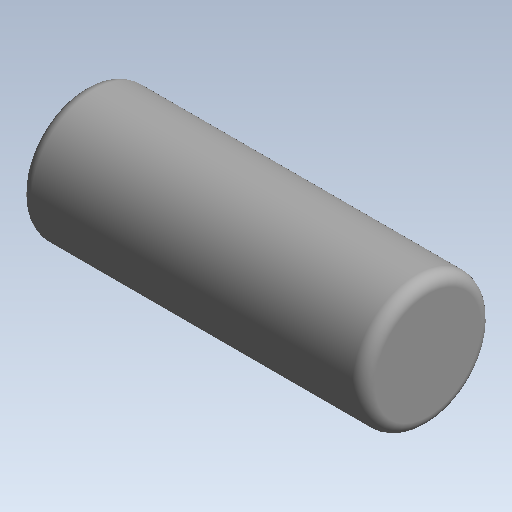
# Autodesk Inventor part: HK0408FT2RO
Saved by Autodesk Inventor 2021.3 (Build 253353010, 353A)
## iProperties
Category: PARTsolutions
Company: NTN
Part Number: HK0408FT2RO
Material: 一般
Catalog Web Link: www.cadenas.de
Description: Needle Roller Shell Bearings open-ended RO-
Vendor: NTN
Document SubType Name: Modeling
Designer: partserver
Manufacturer: NTN
Mass: 0.00703405 g
Surface Area: 0.218287 cm^2
Volume: 0.00703405 cm^3
Density: 1 g/cm^3
Appearance: PSOLRGB-192-192-192
PSOL_IDENT_0: {$CADENAS_DATA\23d-libs\ntn\needle_roler_bearings\needle_roller_shell_bearings_open_ended_ro.prj},19
PSOL_IDENT_1: 8 {VTYP=3D},{NB=HK0408FT2RO},{LINA=HK0408FT2RO},{NN=Needle Roller Shell Bearings open-ended RO},{DAT
PSOL_IDENT_2: E=23.10.2020 01:12:34},{GEOMDATE=20.04.2020 08:34:27},{VERSION=},{LINEID=20},{WBVAR=},{WBNUMERIC=}
PSOL_IDENT_3: {NB=HK0408FT2RO},{LINA=HK0408FT2RO},{KT=DUMMY},{FW=4},{D=8.0},{C=8},{ORDER=HK0408FT2},{CR=1770},{COR=
PSOL_IDENT_4: 1270},{CRF=180},{CORF=129},{LSG=30000},{LSO=45000},{MASS=0.0016},{IT=-},{RT=1.6},{VER=1},{T=0.500},{
PSOL_IDENT_5: DW=1.500},{LW=4.000},{NR=6.000},{CID=4.750},{CD=6.250},{CW=6.600},{SD=4.200}
NB: HK0408FT2RO
NN: Needle Roller Shell Bearings open-ended RO
NBSYN: $ORDER.RO
LINA: HK0408FT2RO
CATALOG: NTN Corporation
FW: 4
D: 8
C: 8
ORDER: HK0408FT2
CR: 1770
COR: 1270
CRF: 180
CORF: 129
LSG: 30000
LSO: 45000
MASS: 0.0016
IT: -
RT: 1.6
VER: 1
SUPPLIER: NTN
ARTICLENO: HK0408FT2RO
BOMINFO: HK0408FT2RO
CREATOR: CADENAS GmbH
Title: HK0408FT2RO
Author: Cadenas PARTsolutions
Autodesk Inventor part; units mm, degrees
sketch "Sketch_1" plane through (0, 0, 0) normal (0, 0, 1) x (1, 0, 0)
  line L0 (2, 0) -> (-2, 0)
  line L1 (-2, 0) -> (-2, 0.6167)
  arc A0 (-1.8667, 0.75) -> (-2, 0.6167) centre (-1.8667, 0.6167) ccw
  line L2 (-1.8667, 0.75) -> (1.8667, 0.75)
  arc A1 (2, 0.6167) -> (1.8667, 0.75) centre (1.8667, 0.6167) ccw
  line L3 (2, 0.6167) -> (2, 0)
  line L4 (2, 0) -> (-2, 0)
  constraints: 10 end point, 4 point on circle, 2 centre point
revolve "Revolution1" add sketch "Sketch_1" angle 360 about axis through (2, 0, 0) along (1, 0, 0)
ref_plane "IP_1_XY" through (0, 0, 0) normal (1, 0, 0) x (0, 0, -1)
ref_plane "IP_1_YZ" through (0, 0, 0) normal (0, 0, -1) x (0, 1, 0)
ref_plane "IP_1_ZX" through (0, 0, 0) normal (0, 1, 0) x (1, 0, 0)
body "Solid1"
